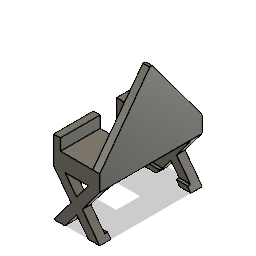
Playground Holder v1 (Autodesk Fusion 360 design; units mm, degrees)
Autodesk Fusion 360 part; units mm, degrees
sketch "Sketch1" plane through (0, 0, 0) normal (0, 1, 0) x (1, 0, 0)
  line L0 (10, 22.225) -> (-10, 22.225)
  line L1 (-10, 22.225) -> (-10, -22.225)
  line L2 (-10, -22.225) -> (10, -22.225)
  line L3 (10, -22.225) -> (10, 22.225)
  line L4 (10, 22.225) -> (-10, -22.225) construction
  line L5 (-10, 22.225) -> (10, -22.225) construction
  dimension "d1" = 44.45
  dimension "d2" = 20
extrude "Extrude1" add sketch "Sketch1" along normal blind 7
sketch "Sketch2" plane through (0, 7, 0) normal (0, 1, 0) x (-1, 0, 0)
  line L0 (-10, 22.225) -> (-10, -22.225)
  line L1 (-10, -22.225) -> (10, -22.225)
  line L2 (10, -22.225) -> (10, 22.225)
  line L3 (10, 22.225) -> (-10, 22.225)
  line L4 (10, -22.225) -> (7, -22.225)
  line L5 (7, -22.225) -> (7, 22.225)
  line L6 (7, 22.225) -> (10, 22.225)
  line L7 (10, 22.225) -> (10, -22.225)
  dimension "d5" = 44.45
  dimension "d6" = 3
extrude "Extrude2" add sketch "Sketch2" along normal blind 5 contours L1 L2 L3 L4 L5 L6 L7
sketch "Sketch3" plane through (0, 7, 0) normal (0, 1, 0) x (-1, 0, 0)
  line L0 (7, -22.225) -> (7, 22.225)
  line L1 (7, 22.225) -> (-10, 22.225)
  line L2 (-10, 22.225) -> (-10, -22.225)
  line L3 (-10, -22.225) -> (7, -22.225)
  line L4 (-10, -22.225) -> (-7, -22.225)
  line L5 (-7, -22.225) -> (-7, 22.225)
  line L6 (-7, 22.225) -> (-10, 22.225)
  line L7 (-10, 22.225) -> (-10, -22.225)
  dimension "d9" = 44.45
  dimension "d10" = 3
extrude "Extrude3" add sketch "Sketch3" along normal blind 30 contours L1 L2 L3 L4 L5 L6 L7
sketch "Sketch4" plane through (-10, 0, 0) normal (-1, 0, 0) x (0, 0, 1)
  line L0 (-22.225, 0) -> (22.225, 0)
  line L1 (22.225, 0) -> (22.225, 12)
  line L2 (22.225, 12) -> (-22.225, 12)
  line L3 (-22.225, 12) -> (-22.225, 0)
  line L4 (-5, 0) -> (5, 0)
  line L5 (5, 0) -> (5, 12)
  line L6 (5, 12) -> (-5, 12)
  line L7 (-5, 12) -> (-5, 0)
extrude "Extrude4" cut sketch "Sketch4" against normal blind 10 contours L0 L2 L4 L5 L6 L7
sketch "Sketch5" plane through (7, 0, 0) normal (-1, 0, 0) x (0, 0, 1)
  line L0 (-22.225, 7) -> (22.225, 7)
  line L1 (22.225, 7) -> (22.225, 37)
  line L2 (22.225, 37) -> (-22.225, 37)
  line L3 (-22.225, 37) -> (-22.225, 7)
  line L4 (-22.225, 7) -> (0, 37)
  line L5 (0, 37) -> (22.225, 7)
  line L6 (-22.225, 7) -> (22.225, 7)
extrude "Extrude5" cut sketch "Sketch5" against normal blind 3 contours L2 L3 L4 | L1 L2 L5
sketch "Sketch6" plane through (0, 0, 0) normal (0, -1, 0) x (1, 0, 0)
  line L0 (0, -5) -> (-10, -5)
  line L1 (-10, -5) -> (-10, -22.225)
  line L2 (-10, -22.225) -> (10, -22.225)
  line L3 (10, -22.225) -> (10, 22.225)
  line L4 (10, 22.225) -> (-10, 22.225)
  line L5 (-10, 22.225) -> (-10, 5)
  line L6 (-10, 5) -> (0, 5)
  line L7 (0, 5) -> (0, -5)
  line L8 (-10, -22.225) -> (-5, -22.225)
  line L9 (-5, -22.225) -> (-5, -17.225)
  line L10 (-5, -17.225) -> (-10, -17.225)
  line L11 (-10, -17.225) -> (-10, -22.225)
  line L12 (10, -22.225) -> (5, -22.225)
  line L13 (5, -22.225) -> (5, -17.225)
  line L14 (5, -17.225) -> (10, -17.225)
  line L15 (10, -17.225) -> (10, -22.225)
  line L16 (-22, 0) -> (28, 0) construction
  line L17 (-5, 17.225) -> (-10, 17.225)
  line L18 (-5, 22.225) -> (-5, 17.225)
  line L19 (-10, 22.225) -> (-5, 22.225)
  line L20 (-10, 17.225) -> (-10, 22.225)
  line L21 (5, 17.225) -> (10, 17.225)
  line L22 (5, 22.225) -> (5, 17.225)
  line L23 (10, 22.225) -> (5, 22.225)
  line L24 (10, 17.225) -> (10, 22.225)
  dimension "d17" = 5
  dimension "d18" = 5
  dimension "d19" = 5
  dimension "d20" = 5
sketch "Sketch7" plane through (0, 0, -22.225) normal (0, 0, -1) x (-1, 0, 0)
  line L0 (-7, 7) -> (-10, 7)
  line L1 (-10, 7) -> (-10, 0)
  line L2 (-10, 0) -> (10, 0)
  line L3 (10, 0) -> (10, 12)
  line L4 (10, 12) -> (7, 12)
  line L5 (7, 12) -> (7, 7)
  line L6 (7, 7) -> (-7, 7)
  line L7 (5, 0) -> (5, -31) construction
  line L8 (-5, 0) -> (-5, -31) construction
  line L9 (-10, 0) -> (5, -20)
  line L10 (10, 0) -> (-5, -20)
sweep "Sweep3" add profiles "Sketch6" path "Sketch7" along L10 section 1 contours L1 L2 L8 L9 L10 L11 | L4 L5 L17 L18 L19 L20
sweep "Sweep4" add profiles "Sketch6" path "Sketch7" along L9 section 1 contours L2 L3 L12 L13 L14 L15 | L3 L4 L21 L22 L23 L24
sketch "Sketch9" plane through (0, -20, 0) normal (0, -1, 0) x (1, 0, 0)
  line L0 (5, -17.225) -> (5, -22.225)
  line L1 (5, -22.225) -> (10, -22.225)
  line L2 (10, -22.225) -> (10, -17.225)
  line L3 (10, -17.225) -> (5, -17.225)
  line L4 (-10, -22.225) -> (10, 22.225) construction
  line L5 (10, 22.225) -> (-10, 22.225) construction
  line L6 (-10, 22.225) -> (10, -22.225) construction
sketch "Sketch10" plane through (-10, 0, 0) normal (-1, 0, 0) x (0, 0, 1)
  line L0 (-5, 0) -> (-5, 12)
  line L1 (-5, 12) -> (-22.225, 12)
  line L2 (-22.225, 12) -> (-22.225, 0)
  line L3 (-22.225, 0) -> (-17.225, 0)
  line L4 (-17.225, 0) -> (-5, 0)
  line L5 (18.5, -2) -> (-18.5, -2)
  line L6 (-18.5, -2) -> (-18.5, -18)
  line L7 (-18.5, -18) -> (18.5, -18)
  line L8 (18.5, -18) -> (18.5, -2)
  line L9 (18.5, -2) -> (-18.5, -18) construction
  line L10 (-18.5, -2) -> (18.5, -18) construction
  dimension "d56" = 37
  dimension "d57" = 16
extrude "Extrude6" cut sketch "Sketch10" against normal blind 21 contours L5 L6 L7 L8
sketch "Sketch11" plane through (0, 0, 0) normal (0, -1, 0) x (1, 0, 0)
  line L0 (-3.9365, -21.2238) -> (3.4775, -21.2238) construction
  line L1 (3.4775, -21.2238) -> (3.4775, -19.2238) construction
  line L2 (3.4775, -19.2238) -> (-3.9365, -19.2238) construction
  line L3 (-3.9365, -19.2238) -> (-3.9365, -21.2238) construction
  text T0 "H.S v1.0" font "Arial" height 2 align ink ink in box 0 x 0 at (-3.9365, -21.2238) x (1, 0) y (0, 1) spacing 1 height is em
extrude "Extrude7" cut sketch "Sketch11" against normal blind 0.2 text T0
chamfer "Chamfer1" distance 1 angle 45 1 edges at (8.5, 37, 0)
